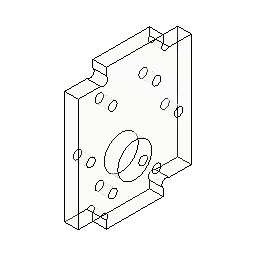
AssemblyMotor v7 (Autodesk Fusion 360 archive; units mm, degrees)
design "MotorDocking40"
Autodesk Fusion 360 part; units mm, degrees
sketch "Sketch1" plane through (0, 0, 0) normal (1, 0, 0) x (0, 1, 0)
  line L0 (-20, 20) -> (20, 20) construction
  line L1 (20, 20) -> (20, -20)
  line L2 (20, -20) -> (-20, -20) construction
  line L3 (-20, -20) -> (-20, 20)
  line L4 (0, 0) -> (0, 20) construction
  line L5 (0, 0) -> (20, 0) construction
  line L6 (0, 0) -> (0, -1.6) construction
  line L7 (0, 0) -> (0, -8.6) construction
  circle A0 centre (0, -8.6) radius 6
  circle A1 centre (0, -1.6) radius 18.4 construction
  circle A2 centre (0, -1.6) radius 15.5 construction
  line L8 (0, -1.6) -> (15.5, -1.6) construction
  circle A3 centre (15.5, -1.6) radius 1.5
  circle A4 centre (7.75, 11.8234) radius 1.5
  circle A5 centre (-7.75, 11.8234) radius 1.5
  circle A6 centre (-15.5, -1.6) radius 1.5
  circle A7 centre (-7.75, -15.0234) radius 1.5
  circle A8 centre (7.75, -15.0234) radius 1.5
  line L9 (-10, 20) -> (-10, 24.8) construction
  line L10 (-10, 24.8) -> (10, 24.8)
  line L11 (10, 24.8) -> (10, 20) construction
  line L12 (-10, -20) -> (-10, -24.8) construction
  line L13 (-10, -24.8) -> (10, -24.8)
  line L14 (10, -24.8) -> (10, -20) construction
  line L15 (-11.0607, -21.0607) -> (-10, -20) construction
  line L16 (11.0607, -21.0607) -> (10, -20) construction
  line L17 (-11.0607, 21.0607) -> (-10, 20) construction
  line L18 (11.0607, 21.0607) -> (10, 20) construction
  arc A9 (-12.1213, 20) -> (-10, 22.1213) centre (-11.0607, 21.0607) ccw
  arc A10 (-10, 22.1213) -> (-12.1213, 20) centre (-11.0607, 21.0607) ccw construction
  arc A11 (10, 22.1213) -> (12.1213, 20) centre (11.0607, 21.0607) ccw
  arc A12 (12.1213, 20) -> (10, 22.1213) centre (11.0607, 21.0607) ccw construction
  arc A13 (12.1213, -20) -> (10, -22.1213) centre (11.0607, -21.0607) ccw
  arc A14 (10, -22.1213) -> (12.1213, -20) centre (11.0607, -21.0607) ccw construction
  arc A15 (-10, -22.1213) -> (-12.1213, -20) centre (-11.0607, -21.0607) ccw
  arc A16 (-12.1213, -20) -> (-10, -22.1213) centre (-11.0607, -21.0607) ccw construction
  line L19 (-10, 22.1213) -> (-10, 24.8)
  line L20 (-12.1213, 20) -> (-20, 20)
  line L21 (10, 22.1213) -> (10, 24.8)
  line L22 (12.1213, 20) -> (20, 20)
  line L23 (10, -22.1213) -> (10, -24.8)
  line L24 (12.1213, -20) -> (20, -20)
  line L25 (-10, -22.1213) -> (-10, -24.8)
  line L26 (-12.1213, -20) -> (-20, -20)
  dimension "d61" = 40
  dimension "d62" = 40
  dimension "d63" = 1.6
  dimension "d65" = 12
  dimension "d66" = 36.8
  dimension "d67" = 31
  dimension "d68" = 3
  dimension "d70" = 360
  dimension "d71" = 4.8
  dimension "d72" = 20
  dimension "d73" = 10
  dimension "d74" = 4.8
  dimension "d75" = 20
  dimension "d76" = 10
  dimension "d77" = 3
  dimension "d78" = 1.5
  dimension "d79" = 45
  dimension "d80" = 3
  dimension "d81" = 1.5
  dimension "d83" = 45
  dimension "d84" = 3
  dimension "d85" = 3
  dimension "d86" = 1.5
  dimension "d87" = 45
  dimension "d88" = 1.5
  dimension "d89" = 45
  dimension "d90" = 7
  constraint horizontal L0
  constraint vertical L1
  constraint horizontal L2
  constraint vertical L3
  constraint coincident L4.start L5.start
  constraint midpoint L0 L4.end
  constraint midpoint L1 L5.end
  constraint vertical L4
  constraint horizontal L5
  constraint perpendicular L5 L6
  constraint perpendicular L5 L7
  constraint coincident L7.end A0.centre
  constraint coincident L6.end A1.centre
  constraint concentric A1 A2
  constraint coincident A2 L8.end
  constraint perpendicular L6 L8
  constraint coincident L8.end A3.centre
  constraint coincident L0 L9.start
  constraint perpendicular L0 L9
  constraint perpendicular L9 L10
  constraint coincident L0 L11.end
  constraint perpendicular L0 L11
  constraint coincident L2 L12.start
  constraint perpendicular L2 L12
  constraint perpendicular L12 L13
  constraint coincident L2 L14.end
  constraint perpendicular L2 L14
  constraint coincident L15.start A15.centre
  constraint coincident L16.start A13.centre
  constraint coincident L17.start A9.centre
  constraint coincident L18.start A11.centre
  constraint coincident L9 A9.end
  constraint coincident L0 A9.start
  constraint concentric A9 A10
  constraint coincident L0 A11.end
  constraint coincident L11 A11.start
  constraint concentric A11 A12
  constraint coincident L14 A13.end
  constraint coincident L2 A13.start
  constraint concentric A13 A14
  constraint coincident L2 A15.end
  constraint coincident L12 A15.start
  constraint concentric A15 A16
  measures "d61" distance of L0.start L2.end
  measures "d62" distance of L0.start L0.end
  measures "d63" distance of L4.start L6.end
  measures "d65" diameter of A0
  measures "d66" diameter of A1
  measures "d67" diameter of A2
  measures "d68" diameter of A3
  measures "d71" distance of L9.start L9.end
  measures "d72" distance of L9.end L10.end
  measures "d73" distance of L3 L9
  measures "d74" distance of L12.start L12.end
  measures "d75" distance of L12.end L13.end
  measures "d76" distance of L3 L12
  measures "d77" diameter of A15
  measures "d78" distance of L12.start L15.start
  measures "d79" angle of L2 L15
  measures "d80" diameter of A13
  measures "d81" distance of L14.end L16.start
  measures "d83" angle of L2 L16
  measures "d84" diameter of A11
  measures "d85" diameter of A9
  measures "d86" distance of L11.end L18.start
  measures "d87" angle of L0 L18
  measures "d88" distance of L9.start L17.start
  measures "d89" angle of L0 L17
  measures "d90" distance of L7.end L6.end
extrude "Extrude1" add sketch "Sketch1" along normal blind 4.8

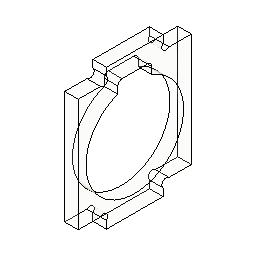
design "MotorDockBack40"
Autodesk Fusion 360 part; units mm, degrees
sketch "Sketch1" plane through (0, 0, 0) normal (1, 0, 0) x (0, 1, 0)
  line L0 (-20, 20) -> (20, 20) construction
  line L1 (20, 20) -> (20, -20)
  line L2 (20, -20) -> (-20, -20) construction
  line L3 (-20, -20) -> (-20, 20)
  line L4 (0, 0) -> (20, 0) construction
  line L5 (0, 0) -> (0, 20) construction
  line L6 (-10, 20) -> (-10, 24.8) construction
  line L7 (-10, 24.8) -> (10, 24.8)
  line L8 (10, 24.8) -> (10, 20) construction
  line L9 (-10, -20) -> (-10, -24.8) construction
  line L10 (-10, -24.8) -> (10, -24.8)
  line L11 (10, -24.8) -> (10, -20) construction
  line L12 (0, 0) -> (0, -1.6) construction
  line L13 (-6, 17.0729) -> (-6, 18.5729) construction
  line L14 (-6, 18.5729) -> (6, 18.5729) construction
  line L15 (6, 18.5729) -> (6, 17.0729) construction
  line L16 (-11.0607, 21.0607) -> (-10, 20) construction
  line L17 (11.0607, 21.0607) -> (10, 20) construction
  line L18 (11.0607, -21.0607) -> (10, -20) construction
  line L19 (-11.0607, -21.0607) -> (-10, -20) construction
  arc A0 (-6, 17.0729) -> (-4.5, 18.5729) centre (-4.5, 17.0729) ccw construction
  arc A1 (-4.5, 18.5729) -> (-6, 17.0729) centre (-4.5, 17.0729) ccw
  arc A2 (4.5, 18.5729) -> (6, 17.0729) centre (4.5, 17.0729) ccw construction
  arc A3 (6, 17.0729) -> (4.5, 18.5729) centre (4.5, 17.0729) ccw
  line L20 (-6, 14.5729) -> (-6, 17.0729)
  line L21 (6, 17.0729) -> (6, 14.5729)
  arc A4 (-6, 14.5729) -> (6, 14.5729) centre (0, -1.6) ccw
  arc A5 (6, 14.5729) -> (0, 15.65) centre (0, -1.6) ccw construction
  arc A6 (0, 15.65) -> (-6, 14.5729) centre (0, -1.6) ccw construction
  line L22 (-4.5, 18.5729) -> (4.5, 18.5729)
  arc A7 (-12.1213, 20) -> (-10, 22.1213) centre (-11.0607, 21.0607) ccw
  arc A8 (-10, 22.1213) -> (-12.1213, 20) centre (-11.0607, 21.0607) ccw construction
  arc A9 (10, 22.1213) -> (12.1213, 20) centre (11.0607, 21.0607) ccw
  arc A10 (12.1213, 20) -> (10, 22.1213) centre (11.0607, 21.0607) ccw construction
  arc A11 (-10, -22.1213) -> (-12.1213, -20) centre (-11.0607, -21.0607) ccw
  arc A12 (-12.1213, -20) -> (-10, -22.1213) centre (-11.0607, -21.0607) ccw construction
  arc A13 (12.1213, -20) -> (10, -22.1213) centre (11.0607, -21.0607) ccw
  arc A14 (10, -22.1213) -> (12.1213, -20) centre (11.0607, -21.0607) ccw construction
  line L23 (-10, 22.1213) -> (-10, 24.8)
  line L24 (10, 22.1213) -> (10, 24.8)
  line L25 (12.1213, 20) -> (20, 20)
  line L26 (-12.1213, 20) -> (-20, 20)
  line L27 (-20, -20) -> (-12.1213, -20)
  line L28 (-10, -22.1213) -> (-10, -24.8)
  line L29 (10, -22.1213) -> (10, -24.8)
  line L30 (12.1213, -20) -> (20, -20)
  point P0 (0, 18.5729)
  dimension "d39" = 40
  dimension "d40" = 40
  dimension "d41" = 4.8
  dimension "d42" = 20
  dimension "d43" = 10
  dimension "d44" = 4.8
  dimension "d45" = 20
  dimension "d46" = 10
  dimension "d47" = 1.6
  dimension "d48" = 34.5
  dimension "d49" = 4
  dimension "d51" = 3
  dimension "d52" = 1.5
  dimension "d53" = 45
  dimension "d54" = 3
  dimension "d55" = 3
  dimension "d56" = 3
  dimension "d57" = 1.5
  dimension "d58" = 45
  dimension "d59" = 3
  dimension "d60" = 1.5
  dimension "d61" = 45
  dimension "d62" = 3
  dimension "d63" = 1.5
  dimension "d64" = 45
  dimension "d65" = 12
  constraint horizontal L0
  constraint vertical L1
  constraint horizontal L2
  constraint vertical L3
  constraint coincident L4.start L5.start
  constraint midpoint L1 L4.end
  constraint midpoint L0 L5.end
  constraint horizontal L4
  constraint vertical L5
  constraint coincident L0 L6.start
  constraint perpendicular L0 L6
  constraint perpendicular L6 L7
  constraint coincident L0 L8.end
  constraint perpendicular L0 L8
  constraint coincident L2 L9.start
  constraint perpendicular L2 L9
  constraint perpendicular L9 L10
  constraint coincident L2 L11.end
  constraint perpendicular L2 L11
  constraint perpendicular L4 L12
  constraint coincident L12.end A4.centre
  constraint perpendicular L0 L13
  constraint perpendicular L5 L14
  constraint perpendicular L14 L15
  constraint midpoint L14 P0
  constraint coincident L5 P0
  constraint coincident L16.start A7.centre
  constraint tangent L14 A0
  constraint tangent L13 A0
  constraint tangent L14 A2
  constraint tangent L15 A2
  constraint coincident L17.start A9.centre
  constraint coincident L18.start A13.centre
  constraint coincident L19.start A11.centre
  constraint coincident L14 A0.end
  constraint concentric A0 A1
  constraint coincident L14 A2.start
  constraint concentric A2 A3
  constraint perpendicular L0 L20
  constraint perpendicular L14 L21
  constraint coincident L5 A5.end
  constraint concentric A4 A5
  constraint concentric A4 A6
  constraint coincident L6 A7.end
  constraint coincident L0 A7.start
  constraint concentric A7 A8
  constraint coincident L0 A9.end
  constraint coincident L8 A9.start
  constraint concentric A9 A10
  constraint coincident L2 A11.end
  constraint coincident L9 A11.start
  constraint concentric A11 A12
  constraint coincident L11 A13.end
  constraint coincident L2 A13.start
  constraint concentric A13 A14
  measures "d39" distance of L0.start L0.end
  measures "d40" distance of L0.start L2.end
  measures "d41" distance of L6.start L6.end
  measures "d42" distance of L6.end L7.end
  measures "d43" distance of L3 L6
  measures "d44" distance of L9.start L9.end
  measures "d45" distance of L9.end L10.end
  measures "d46" distance of L3 L9
  measures "d47" distance of L4.start L12.end
  measures "d48" diameter of A4
  measures "d49" distance of L20.start L13.end
  measures "d51" diameter of A7
  measures "d52" distance of L6.start L16.start
  measures "d53" angle of L0 L16
  measures "d54" diameter of A0
  measures "d55" diameter of A2
  measures "d56" diameter of A9
  measures "d57" distance of L8.end L17.start
  measures "d58" angle of L0 L17
  measures "d59" diameter of A13
  measures "d60" distance of L11.end L18.start
  measures "d61" angle of L2 L18
  measures "d62" diameter of A11
  measures "d63" distance of L9.start L19.start
  measures "d64" angle of L2 L19
  measures "d65" distance of L20 L21
extrude "Extrude1" add sketch "Sketch1" along normal blind 4.8
